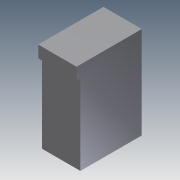
# Autodesk Inventor part: battery
Saved by Autodesk Inventor 2011 (Build 150239000, 239)
## iProperties
Created: 2011-12-30
Part Number: battery
Document SubType Name: Modeling
Designer: Matthew
Density: 1 g/cm^3
Author: Matthew
Autodesk Inventor part; units mm, degrees
ref_plane "YZ Plane" through (0, 0, 0) normal (1, 0, 0) x (0, 1, 0)
ref_plane "XZ Plane" through (0, 0, 0) normal (0, 1, 0) x (-1, 0, 0)
ref_plane "XY Plane" through (0, 0, 0) normal (0, 0, 1) x (1, 0, 0)
sketch "Sketch1" plane through (0, 0, 0) normal (0, 0, 1) x (1, 0, 0)
  line L0 (-38.2565, 12.5) -> (25.2435, 12.5)
  line L1 (25.2435, 12.5) -> (25.2435, -139.9)
  line L2 (25.2435, -139.9) -> (-38.2565, -139.9)
  line L3 (-38.2565, -139.9) -> (-38.2565, 12.5)
  point P0 (0, 0)
  dimension "d0" = 63.5
  dimension "d1" = 152.4
  constraints: 8 end point, 2 parallel, 1 horizontal, 1 perpendicular
  measures "d0" distance of L1.end L2.end
  measures "d1" distance of L0.end L1.end
extrude "Extrusion1" add sketch "Sketch1" along normal blind 114.3
sketch "Sketch2" plane through (0, 0, 114.3) normal (0, 0, 1) x (1, 0, 0)
  line L0 (-38.2565, -139.9) -> (-38.2565, 12.5) projected
  line L1 (25.2435, -139.9) -> (-38.2565, -139.9) projected
  line L2 (-38.2565, -7.0772) -> (25.2435, -7.0772)
  line L3 (25.2435, -7.0772) -> (25.2435, -139.9)
  line L4 (25.2435, -139.9) -> (-38.2565, -139.9)
  line L5 (-38.2565, -139.9) -> (-38.2565, -7.0772)
  point P0 (0, 0)
  constraints: 8 end point, 2 parallel, 1 horizontal, 1 perpendicular, 1 point on line
extrude "Extrusion2" cut sketch "Sketch2" against normal blind 6.35
sketch "Sketch3" plane through (0, 0, 0) normal (0, 0, -1) x (-1, 0, 0)
  line L0 (38.2565, 12.5) -> (-25.2435, 12.5) projected
  line L1 (-25.2435, 12.5) -> (-25.2435, -139.9) projected
  line L2 (-25.2435, -139.9) -> (38.2565, -139.9) projected
  line L3 (38.2565, -139.9) -> (38.2565, 12.5) projected
  point P0 (0, 0)
extrude "Extrusion3" cut sketch "Sketch3" against normal blind 6.35
body "Solid1"
